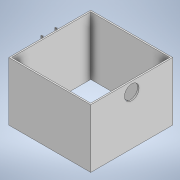
# Autodesk Inventor part: cube bucket new
Saved by Autodesk Inventor 2021 (Build 250183000, 183)
## iProperties
Created: 2021-07-23
Part Number: cube bucket new
Material: Generic
Document SubType Name: Modeling
Designer: Nishat
Density: 1 g/cm^3
Appearance: Default
Mass: 1.09056e+06 g
Surface Area: 448259 cm^2
Volume: 1.09056e+06 cm^3
Author: Nishat
Autodesk Inventor part; units mm, degrees
ref_plane "YZ Plane" through (0, 0, 0) normal (1, 0, 0) x (0, 1, 0)
ref_plane "XZ Plane" through (0, 0, 0) normal (0, 1, 0) x (-1, 0, 0)
ref_plane "XY Plane" through (0, 0, 0) normal (0, 0, 1) x (1, 0, 0)
sketch "Sketch1" plane through (0, 0, 0) normal (0, 1, 0) x (-1, 0, 0)
  line L0 (1400, 1400) -> (-1400, 1400)
  line L1 (-1400, 1400) -> (-1400, -1400)
  line L2 (-1400, -1400) -> (1400, -1400)
  line L3 (1400, -1400) -> (1400, 1400)
  point P0 (0, 0)
  dimension "d0" = 2800
  dimension "d1" = 2800
  dimension "d2" = 1400
  dimension "d3" = 1400
  constraints: 8 end point, 2 parallel, 1 horizontal, 1 perpendicular
  measures "d0" distance between parallel lines of L1 L3
  measures "d1" distance between parallel lines of L2 L0
  measures "d2" distance from line of L0 point (0, 0)
  measures "d3" distance from line of point (0, 0) L3
extrude "Extrusion1" add sketch "Sketch1" along normal blind 2000
sketch "Sketch2" plane through (1400, 0, 1400) normal (1, 0, 0) x (0, 0, -1)
  circle A0 centre (1400, 1671.5944) radius 250
  point P0 (1400, 0)
  dimension "d6" = 500
  constraints: 1 centre point
  measures "d6" diameter of A0
extrude "Extrusion2" cut sketch "Sketch2" against normal blind 2000
sketch "Sketch3" plane through (0, 2000, 0) normal (0, 1, 0) x (1, 0, 0)
  line L0 (-1350, -1350) -> (1350, -1350)
  line L1 (1350, -1350) -> (1350, 1350)
  line L2 (1350, 1350) -> (-1350, 1350)
  line L3 (-1350, 1350) -> (-1350, -1350)
  point P0 (0, 0)
  dimension "d9" = 2700
  dimension "d10" = 2700
  dimension "d11" = 1350
  dimension "d12" = 1350
  constraints: 8 end point, 2 parallel, 1 horizontal, 1 perpendicular
  measures "d9" distance between parallel lines of L1 L3
  measures "d10" distance between parallel lines of L2 L0
  measures "d11" distance from line of L3 point (0, 0)
  measures "d12" distance from line of point (0, 0) L0
extrude "Extrusion3" cut sketch "Sketch3" against normal blind 2000
sketch "Sketch7" plane through (-1400, 0, -1400) normal (-1, 0, 0) x (0, 0, 1)
  line L0 (2800, 2000) -> (0, 2000) projected
  line L1 (1650, 1900) -> (1150, 1900)
  line L2 (1150, 1900) -> (1150, 2000)
  line L3 (1150, 2000) -> (1650, 2000)
  line L4 (1650, 2000) -> (1650, 1900)
  line L5 (2800, 0) -> (2800, 2000) projected
  line L6 (2750, 2000) -> (50, 2000) projected
  line L7 (1625, 1900) -> (1175, 1900)
  line L8 (1175, 1900) -> (1175, 2000)
  line L9 (1175, 2000) -> (1625, 2000)
  line L10 (1625, 2000) -> (1625, 1900)
  point P0 (1400, 0)
  dimension "d22" = 500
  dimension "d23" = 1150
  dimension "d24" = 100
  dimension "d25" = 450
  dimension "d26" = 25
  constraints: 16 end point, 4 parallel, 3 point on line, 2 horizontal, 2 perpendicular
  measures "d22" distance between parallel lines of L2 L4
  measures "d23" distance between parallel lines of L4 L5
  measures "d24" distance between parallel lines of L1 L0
  measures "d25" distance between parallel lines of L8 L10
  measures "d26" distance between parallel lines of L10 L4
sketch "Sketch8" plane through (-1400, 0, -1400) normal (-1, 0, 0) x (0, 0, 1)
  line L0 (2800, 2000) -> (0, 2000) projected
  line L1 (1174.764, 1899.7185) -> (1150.0977, 1899.7185)
  line L2 (1150.0977, 1899.7185) -> (1150.0977, 2000)
  line L3 (1150.0977, 2000) -> (1174.764, 2000)
  line L4 (1174.764, 2000) -> (1174.764, 1899.7185)
  point P0 (1400, 0)
  constraints: 8 end point, 2 parallel, 1 horizontal, 1 perpendicular, 1 point on line
extrude "Extrusion7" add sketch "Sketch7" along normal blind 50 contours L4 L1 L10 L0
extrude "Extrusion8" add sketch "Sketch8" along normal blind 50
sketch "Sketch10" plane through (0, 2000, 0) normal (0, 1, 0) x (1, 0, 0)
  line L0 (-1400, -250) -> (-1450, -250) projected
  line L1 (-1400, -225) -> (-1450, -225) projected
  line L2 (-1450, -250) -> (-1400, -250)
  line L3 (-1400, -250) -> (-1400, -225)
  line L4 (-1400, -225) -> (-1450, -225)
  line L5 (-1450, -225) -> (-1450, -250)
  line L6 (-1400, 225.236) -> (-1450, 225.236) projected
  line L7 (-1400, 1400) -> (-1400, -1400) projected
  line L8 (-1450, 225.236) -> (-1400, 225.236)
  line L9 (-1400, 225.236) -> (-1400, 250.2305)
  line L10 (-1400, 250.2305) -> (-1450, 250.2305)
  line L11 (-1450, 250.2305) -> (-1450, 225.236)
  point P0 (0, 0)
  constraints: 16 end point, 4 parallel, 2 horizontal, 2 perpendicular, 1 point on line
extrude "Extrusion9" add sketch "Sketch10" along normal blind 50
sketch "Sketch11" plane through (-1450, 1900, 250) normal (0, 0, 1) x (1, 0, 0)
  circle A0 centre (25, 125) radius 15
  line L0 (50, 100) -> (50, 150) projected
  point P0 (1450, -1900)
  dimension "d33" = 30
  dimension "d34" = 10
  constraints: 1 centre point
  measures "d33" diameter of A0
  measures "d34" distance edge to line of A0 L0
extrude "Extrusion10" cut sketch "Sketch11" against normal blind 700
body "Solid1"
